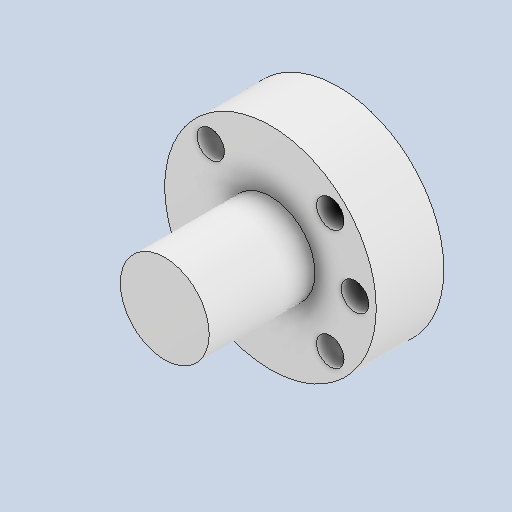
# Autodesk Inventor part: BaseImpresion
Saved by Autodesk Inventor 2023 (Build 270158000, 158)
## iProperties
Created: 2022-08-25
Part Number: BaseImpresion
Material: PVC-Piping
Document SubType Name: Modeling
Designer: andre
Density: 1.4 g/cm^3
Appearance: Smooth - White
Mass: 36.6153 g
Surface Area: 93.1286 cm^2
Volume: 36.6153 cm^3
Author: andre
Autodesk Inventor part; units mm, degrees
ref_plane "YZ Plane" through (0, 0, 0) normal (1, 0, 0) x (0, 1, 0)
ref_plane "XZ Plane" through (0, 0, 0) normal (0, 1, 0) x (-1, 0, 0)
ref_plane "XY Plane" through (0, 0, 0) normal (0, 0, 1) x (1, 0, 0)
sketch "Sketch1" plane through (0, 0, 0) normal (0, 0, 1) x (1, 0, 0)
  circle A0 centre (0, 0) radius 25
  line L0 (0, 0) -> (20, 0) construction
  dimension "d0" = 50
  dimension "d1" = 20
  constraints: 2 end point, 1 centre point, 1 coincident, 1 horizontal
  measures "d0" diameter of A0
  measures "d1" distance of L0.start L0.end
extrude "Extrusion1" add sketch "Sketch1" along normal blind 16
sketch "Sketch2" plane through (0, 0, 16) normal (0, 0, 1) x (1, 0, 0)
  circle A0 centre (0, 0) radius 25 projected
  point P0 (-14.1421, 14.1421)
  point P1 (-14.1421, -14.1421)
  point P2 (14.1421, -14.1421)
  point P3 (14.1421, 14.1421)
  dimension "d18" = 360
  constraints: 5 other
hole "Hole1" at (-14.1421, 14.1421, 16) at (-14.1421, -14.1421, 16) at (14.1421, -14.1421, 16) at (14.1421, 14.1421, 16) direction (0, 0, -1) diameter 6.5 end through all
sketch "Sketch11" plane through (0, 0, 16) normal (0, 0, 1) x (1, 0, 0)
  line L0 (0, 0) -> (20, 0)
  dimension "d68" = 20
  constraints: 2 end point, 1 coincident, 1 horizontal
  measures "d68" distance of L0.start L0.end
hole "Hole4" at (20, 0, 16) direction (0, 0, -1) diameter 6.5 end through all
sketch "Sketch12" plane through (0, 0, 16) normal (0, 0, 1) x (1, 0, 0)
  circle A0 centre (0, 0) radius 10.5
  dimension "d76" = 21
  constraints: 1 centre point, 1 coincident
  measures "d76" diameter of A0
extrude "Extrusion7" add sketch "Sketch12" along normal blind 25
body "Solid1"
